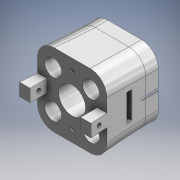
# Autodesk Inventor part: AA008d
Saved by Autodesk Inventor 2017 SP1 (Build 210196100, 196)
## iProperties
Created: 2017-09-28
Part Number: AA008d
Material: ABS Plastic
Document SubType Name: Modeling
Designer: Zach
Density: 1.06 g/cm^3
Appearance: CR White
Author: Zach
Autodesk Inventor part; units mm, degrees
ref_plane "XZ Plane" through (0, 0, 0) normal (0, 1, 0) x (-1, 0, 0)
ref_plane "XY Plane" through (0, 0, 0) normal (0, 0, 1) x (1, 0, 0)
sketch "Sketch1" plane through (0, 0, 0) normal (0, 0, 1) x (1, 0, 0)
  line L0 (0, 0) -> (80, 0)
  line L1 (80, 0) -> (80, 82.6)
  line L2 (80, 82.6) -> (0, 82.6)
  line L3 (0, 82.6) -> (0, 0)
  dimension "d0" = 80
  dimension "d1" = 82.6
  constraints: 8 end point, 2 parallel, 1 horizontal, 1 perpendicular
  measures "d0" distance of L2.end L1.end
  measures "d1" distance of L1.end L0.end
extrude "Extrusion1" add sketch "Sketch1" along normal blind 162.5
sketch "Sketch2" plane through (0, 82.6, 0) normal (0, 1, 0) x (1, 0, 0)
  line L0 (0, -162.5) -> (80, -162.5) projected
  line L1 (-12.5, -162.5) -> (0, -162.5)
  line L2 (80, -162.5) -> (92.5, -162.5)
  line L3 (0, 0) -> (80, 0) projected
  line L4 (0, 0) -> (0, -162.5) projected
  line L5 (80, 0) -> (80, -162.5) projected
  arc A0 (-12.5, -162.5) -> (0, 0) centre (-1199.9534, 10.5733) ccw
  arc A1 (80, 0) -> (92.5, -162.5) centre (1279.9534, 10.5733) ccw
  dimension "d4" = 12.5
  dimension "d5" = 12.5
  dimension "d19" = 1200
  dimension "d20" = 1200
  constraints: 4 end point, 4 point on circle, 2 centre point, 1 collinear, 1 parallel
  measures "d4" distance of L1.start L0.start
  measures "d5" distance of L0.end L2.end
  measures "d19" radius of A0
  measures "d20" radius of A1
extrude "Extrusion2" add sketch "Sketch2" against normal blind 82.6 contours L1 A0 L4 | L5 A1 L2
sketch "Sketch5" plane through (0, 0, 0) normal (0, 0, -1) x (-1, 0, 0)
  line L0 (12.5, 0) -> (-92.5, 0)
  line L1 (-92.5, 0) -> (-92.5, 41.3)
  line L2 (-92.5, 41.3) -> (12.5, 41.3)
  line L3 (12.5, 41.3) -> (12.5, 0)
  point P0 (0, 0)
  point P1 (12.5, 20)
  point P2 (-92.5, 20)
  dimension "d22" = 41.3
  constraints: 8 end point, 2 parallel, 2 point on line, 1 horizontal, 1 horizontal alignment, 1 perpendicular
  measures "d22" distance of L0.end L1.end
extrude "Extrusion4" cut sketch "Sketch5" against normal through all
sketch "Sketch8" plane through (0, 0, 0) normal (1, 0, 0) x (0, 1, 0)
  line L0 (82.6, 162.5) -> (93.8, 162.5)
  line L1 (41.3, 162.5) -> (41.3, 0) projected
  line L2 (82.6, 0) -> (41.3, 0) projected
  arc A0 (93.8, 162.5) -> (82.6, 0) centre (2580.9593, -90.5586) ccw
  line L3 (82.6, 162.5) -> (41.3, 162.5) projected
  line L4 (82.6, 162.5) -> (82.6, 0)
  point P0 (0, 0)
  dimension "d32" = 2500
  dimension "d38" = 11.2
  constraints: 4 end point, 2 point on circle, 1 centre point, 1 horizontal, 1 perpendicular
  measures "d32" radius of A0
  measures "d38" distance of L0.start L0.end
extrude "Extrusion6" add sketch "Sketch8" along normal blind 93 and the other way blind 13 contours L0 A0 L4
sketch "Sketch13" plane through (-13, 82.6, 0) normal (0, -1, 0) x (1, 0, 0)
  arc A0 (13, 0) -> (0.5, 162.5) centre (-1186.9534, -10.5733) ccw projected
  line L0 (0, 162.5) -> (0.5, 162.5) projected
  line L1 (0, 0) -> (0, 162.5) projected
  line L2 (13, 0) -> (0, 0) projected
  arc A1 (105.5, 162.5) -> (93, 0) centre (1292.9534, -10.5733) ccw projected
  line L3 (106, 0) -> (93, 0) projected
  line L4 (106, 162.5) -> (106, 0) projected
  line L5 (105.5, 162.5) -> (106, 162.5) projected
  point P0 (13, 0)
extrude "Extrusion9" cut sketch "Sketch13" against normal through all
fillet "Fillet4" radius 20 2 edges at (-3.5176, 86.9111, 81.8462) (83.5176, 86.9111, 81.8462)
sketch "Sketch38" plane through (0, 0, 162.5) normal (0, 0, 1) x (1, 0, 0)
  line L0 (75, 41.3) -> (5, 41.3)
  circle A0 centre (40, 41.3) radius 4.5
  point P0 (0, 0)
  dimension "d117" = 9
  constraints: 2 end point, 1 centre point, 1 midpoint
  measures "d117" diameter of A0
extrude "Extrusion27" cut sketch "Sketch38" against normal through all
ref_plane "Work Plane14" through (0, 0, 152.5) normal (0, 0, 1) x (1, 0, 0)
sketch "Sketch40" plane through (0, 0, 152.5) normal (0, 0, 1) x (1, 0, 0)
  arc A0 (44.5, 41.3) -> (35.5, 41.3) centre (40, 41.3) ccw projected
  circle A1 centre (40, 41.3) radius 11.5
  point P0 (0, 0)
  dimension "d121" = 23
  constraints: 1 centre point, 1 coincident
  measures "d121" diameter of A1
extrude "Extrusion28" cut sketch "Sketch40" against normal blind 9
ref_plane "Work Plane15" through (0, 0, 61.5) normal (0, 0, 1) x (1, 0, 0)
sketch "Sketch41" plane through (0, 0, 61.5) normal (0, 0, 1) x (1, 0, 0)
  arc A0 (44.5, 41.3) -> (35.5, 41.3) centre (40, 41.3) ccw
  circle A1 centre (40, 41.3) radius 11.5
  point P0 (0, 0)
  dimension "d125" = 23
  constraints: 2 centre point, 2 point on circle, 1 coincident
  measures "d125" diameter of A1
extrude "Extrusion29" cut sketch "Sketch41" against normal blind 9
ref_plane "Work Plane16" through (0, 0, 47.5) normal (0, 0, 1) x (1, 0, 0)
sketch "Sketch43" plane through (0, 0, 47.5) normal (0, 0, 1) x (1, 0, 0)
  arc A0 (44.5, 41.3) -> (35.5, 41.3) centre (40, 41.3) ccw
  line L0 (35.5, 41.3) -> (0, 41.3) construction
  line L1 (0, 62.5933) -> (0, 41.3) construction
  spline S0 degree 3 poles (19.9943, 82.6) (17.3915, 82.6) (14.8137, 82.0916) (9.998, 80.1152) (7.8062, 78.6662) (4.1001, 75.0086) (2.6216, 72.8347) (1.0742, 69.2017) (0.6732, 67.9146) (0.1355, 65.2795) (0, 63.9381) (0, 62.5933) knots 0 0 0 0 0.78083 0.78083 1.561665 1.561665 2.342928 2.342928 2.746314 2.746314 3.149743 3.149743 3.149743 3.149743 construction
  line L2 (60.0057, 82.6) -> (19.9943, 82.6) construction
  spline S1 degree 3 poles (80, 62.5933) (80, 65.2007) (79.4908, 67.7832) (77.5113, 72.6059) (76.0606, 74.8001) (72.4005, 78.5072) (70.2269, 79.985) (66.5969, 81.5295) (65.3131, 81.9291) (62.6848, 82.465) (61.3469, 82.6) (60.0057, 82.6) knots 0 0 0 0 0.782215 0.782215 1.563936 1.563936 2.345071 2.345071 2.747441 2.747441 3.149817 3.149817 3.149817 3.149817 construction
  line L3 (80, 41.3) -> (80, 62.5933) construction
  line L4 (80, 41.3) -> (44.5, 41.3) construction
  line L5 (60.0057, 80.6) -> (19.9943, 80.6)
  line L6 (2, 62.5933) -> (2, 43.3)
  line L7 (2, 43.3) -> (33.8153, 43.3) construction
  arc A1 (46.1847, 43.3) -> (33.8153, 43.3) centre (40, 41.3) ccw construction
  line L8 (46.1847, 43.3) -> (78, 43.3) construction
  line L9 (78, 43.3) -> (78, 62.5933)
  line L10 (2, 43.3) -> (2, 41.3)
  line L11 (78, 43.3) -> (78, 41.3)
  line L12 (44.5, 41.3) -> (78, 41.3)
  line L13 (35.5, 41.3) -> (2, 41.3)
  line L14 (5, 41.3) -> (35.5, 41.3)
  arc A2 (44.5, 41.3) -> (35.5, 41.3) centre (40, 41.3) ccw projected
  spline S2 degree 5 poles (78, 62.5933) (77.9999, 65.4195) (77.4463, 68.2457) (76.3377, 70.927) (73.1281, 75.7135) (68.3466, 78.931) (65.6637, 80.0441) (62.8346, 80.5999) (60.0057, 80.6) knots 0 0 0 0 0 0 0.499755 0.499755 0.499755 1 1 1 1 1 1
  spline S3 degree 5 poles (19.9943, 80.6) (17.1686, 80.5999) (14.3427, 80.0454) (11.6625, 78.9348) (6.8791, 75.7206) (3.666, 70.9361) (2.5549, 68.2521) (2.0001, 65.4227) (2, 62.5933) knots 0 0 0 0 0 0 0.499678 0.499678 0.499678 1 1 1 1 1 1
  dimension "d129" = 2
  constraints: 30 end point, 4 point on circle, 3 centre point, 3 parallel, 2 perpendicular, 2 point on line, 1 collinear, 1 horizontal, 1 horizontal alignment, 18 other
  measures "d129" distance between parallel lines of L3 L9
extrude "Extrusion30" cut sketch "Sketch43" against normal blind 35
sketch "Sketch53" plane through (0, 0, 12.5) normal (0, 0, 1) x (1, 0, 0)
  arc A0 (44.5, 41.3) -> (35.5, 41.3) centre (40, 41.3) ccw projected
  circle A1 centre (40, 41.3) radius 2.5 construction
  line L0 (44.5, 41.3) -> (42.5, 41.3)
  line L1 (35.5, 41.3) -> (37.5, 41.3)
  arc A2 (42.5, 41.3) -> (37.5, 41.3) centre (40, 41.3) ccw
  point P0 (0, 0)
  dimension "d163" = 5
  constraints: 4 end point, 4 point on circle, 2 centre point, 1 coincident, 1 concentric, 1 horizontal, 1 point on line
  measures "d163" diameter of A1
extrude "Extrusion39" add sketch "Sketch53" against normal blind 2
sketch "Sketch54" plane through (0, 0, 0) normal (0, 0, -1) x (-1, 0, 0)
  arc A0 (-35.5, 41.3) -> (-44.5, 41.3) centre (-40, 41.3) ccw projected
  circle A1 centre (-40, 41.3) radius 16.5
  point P0 (0, 0)
  dimension "d166" = 33
  constraints: 1 centre point, 1 coincident
  measures "d166" diameter of A1
extrude "Extrusion40" cut sketch "Sketch54" against normal blind 7.5
sketch "Sketch55" plane through (0, 0, 12.5) normal (0, 0, 1) x (1, 0, 0)
  arc A0 (42.5, 41.3) -> (37.5, 41.3) centre (40, 41.3) ccw projected
  circle A1 centre (40, 49.8) radius 2
  point P0 (0, 0)
  dimension "d169" = 4
  dimension "d170" = 8.5
  constraints: 1 centre point, 1 vertical alignment
  measures "d169" diameter of A1
  measures "d170" distance of A0.centre A1.centre
extrude "Extrusion41" cut sketch "Sketch55" against normal through all
sketch "Sketch56" plane through (0, 0, 12.5) normal (0, 0, 1) x (1, 0, 0)
  circle A0 centre (40, 49.8) radius 2 projected
  circle A1 centre (40, 49.8) radius 3.5
  point P0 (0, 0)
  dimension "d173" = 7
  constraints: 1 centre point, 1 coincident
  measures "d173" diameter of A1
extrude "Extrusion42" cut sketch "Sketch56" against normal blind 3
sketch "Sketch63" plane through (0, 0, 47.5) normal (0, 0, -1) x (-1, 0, 0)
  circle A0 centre (-40, 41.3) radius 16 construction
  arc A1 (-24, 41.3) -> (-56, 41.3) centre (-40, 41.3) ccw
  arc A2 (-35.5, 41.3) -> (-44.5, 41.3) centre (-40, 41.3) ccw construction
  line L0 (-2, 41.3) -> (-35.5, 41.3) construction
  line L1 (-2, 41.3) -> (-2, 62.5933) projected
  spline S0 degree 5 poles (-2, 62.5933) (-2.0001, 65.4227) (-2.5549, 68.2521) (-3.666, 70.9361) (-6.8791, 75.7206) (-11.6625, 78.9348) (-14.3427, 80.0454) (-17.1686, 80.5999) (-19.9943, 80.6) knots 0 0 0 0 0 0 0.500322 0.500322 0.500322 1 1 1 1 1 1 projected
  line L2 (-19.9943, 80.6) -> (-60.0057, 80.6) projected
  spline S1 degree 5 poles (-60.0057, 80.6) (-62.8346, 80.5999) (-65.6637, 80.0441) (-68.3466, 78.931) (-73.1281, 75.7135) (-76.3377, 70.927) (-77.4463, 68.2457) (-77.9999, 65.4195) (-78, 62.5933) knots 0 0 0 0 0 0 0.500245 0.500245 0.500245 1 1 1 1 1 1 projected
  line L3 (-78, 62.5933) -> (-78, 41.3) projected
  line L4 (-44.5, 41.3) -> (-78, 41.3) construction
  line L5 (-78, 41.3) -> (-56, 41.3)
  line L6 (-24, 41.3) -> (-2, 41.3)
  point P0 (0, 0)
  dimension "d207" = 32
  constraints: 4 end point, 4 point on circle, 2 centre point, 2 collinear, 1 coincident, 1 concentric, 1 horizontal alignment, 2 other
  measures "d207" diameter of A0
extrude "Extrusion49" add sketch "Sketch63" along normal blind 35
sketch "Sketch65" plane through (0, 0, 0) normal (0, 0, -1) x (-1, 0, 0)
  circle A0 centre (-40, 71.3) radius 2.5
  arc A1 (-35.5, 41.3) -> (-44.5, 41.3) centre (-40, 41.3) ccw projected
  point P0 (0, 0)
  dimension "d214" = 5
  dimension "d215" = 30
  constraints: 1 centre point, 1 vertical alignment
  measures "d214" diameter of A0
  measures "d215" distance of A1.centre A0.centre
extrude "Extrusion51" cut sketch "Sketch65" against normal blind 75
sketch "Sketch66" plane through (0, 0, 0) normal (0, 0, -1) x (-1, 0, 0)
  circle A0 centre (-40, 71.3) radius 6.5
  circle A1 centre (-40, 71.3) radius 2.5 projected
  point P0 (0, 0)
  dimension "d218" = 13
  constraints: 1 centre point, 1 coincident
  measures "d218" diameter of A0
extrude "Extrusion52" cut sketch "Sketch66" against normal blind 35 contours A0 | A1
mirror "Mirror1" about plane through (92.5, 41.3, 0) normal (0, -1, 0)
sketch "Sketch69" plane through (0, 0, 0) normal (0, 1, 0) x (-1, 0, 0)
  line L0 (-35.5, 143.5) -> (-44.5, 143.5) projected
  line L1 (-51.5, 143.5) -> (-28.5, 143.5) projected
  line L2 (-44.5, 152.5) -> (-35.5, 152.5) projected
  line L3 (-28.5, 61.5) -> (-51.5, 61.5) projected
  line L4 (-44.5, 61.5) -> (-35.5, 61.5) projected
  line L5 (-35.5, 52.5) -> (-44.5, 52.5) projected
  line L6 (-51.5, 61.5) -> (-28.5, 61.5)
  line L7 (-28.5, 61.5) -> (-28.5, 52.5)
  line L8 (-28.5, 52.5) -> (-51.5, 52.5)
  line L9 (-51.5, 52.5) -> (-51.5, 61.5)
  line L10 (-51.5, 143.5) -> (-28.5, 143.5)
  line L11 (-28.5, 143.5) -> (-28.5, 152.5)
  line L12 (-28.5, 152.5) -> (-51.5, 152.5)
  line L13 (-51.5, 152.5) -> (-51.5, 143.5)
  point P0 (0, 0)
  point P1 (-40, 52.5)
  point P2 (-40, 152.5)
  constraints: 16 end point, 4 midpoint, 4 parallel, 2 horizontal, 2 perpendicular, 1 point on line
extrude "Extrusion54" cut sketch "Sketch69" along normal blind 41.5 and the other way blind 15
sketch "Sketch71" plane through (0, 0, 0) normal (0, 0, -1) x (-1, 0, 0)
  line L0 (-17.5, 18.8) -> (-62.5, 18.8) construction
  line L1 (-62.5, 18.8) -> (-62.5, 63.8) construction
  line L2 (-62.5, 63.8) -> (-17.5, 63.8) construction
  line L3 (-17.5, 63.8) -> (-17.5, 18.8) construction
  circle A0 centre (-40, 41.3) radius 4.5 construction
  circle A1 centre (-17.5, 18.8) radius 2.5
  circle A2 centre (-62.5, 18.8) radius 2.5
  circle A3 centre (-62.5, 63.8) radius 2.5
  circle A4 centre (-17.5, 63.8) radius 2.5
  point P0 (0, 0)
  point P1 (-17.5, 41.3)
  point P2 (-40, 18.8)
  dimension "d229" = 45
  dimension "d230" = 45
  dimension "d231" = 5
  dimension "d232" = 5
  dimension "d233" = 5
  dimension "d234" = 5
  constraints: 8 end point, 4 centre point, 4 coincident, 2 midpoint, 2 parallel, 1 horizontal, 1 horizontal alignment, 1 perpendicular, 1 vertical alignment
  measures "d229" distance of L1.end L2.end
  measures "d230" distance of L0.end L1.end
  measures "d231" diameter of A1
  measures "d232" diameter of A2
  measures "d233" diameter of A3
  measures "d234" diameter of A4
extrude "Extrusion56" cut sketch "Sketch71" against normal through all
sketch "Sketch72" plane through (0, 0, 162.5) normal (0, 0, 1) x (1, 0, 0)
  circle A0 centre (40, 41.3) radius 4.5 construction
  line L0 (-12.5, 8.6096) -> (-12.5, 73.9904) construction
  spline S0 degree 3 poles (-12.5, 8.6096) (-12.5, 6.0114) (-11.9936, 3.4396) (-10.0229, -1.3365) (-8.5896, -3.495) (-4.9699, -7.1453) (-2.8204, -8.5984) (0.7865, -10.1299) (2.0756, -10.5292) (4.7184, -11.0654) (6.0655, -11.2) (7.4159, -11.2) knots 0 0 0 0 0.779465 0.779465 1.550261 1.550261 2.321978 2.321978 2.725865 2.725865 3.130971 3.130971 3.130971 3.130971 construction
  line L1 (7.4159, -11.2) -> (72.5841, -11.2) construction
  spline S1 degree 3 poles (72.5841, -11.2) (75.222, -11.2) (77.8346, -10.6862) (82.6695, -8.6891) (84.8494, -7.2416) (88.5077, -3.6012) (89.955, -1.4536) (91.9757, 3.3497) (92.5, 5.9658) (92.5, 8.6096) knots 0 0 0 0 0.791372 0.791372 1.569712 1.569712 2.340306 2.340306 3.13363 3.13363 3.13363 3.13363 construction
  line L2 (92.5, 73.9904) -> (92.5, 8.6096) construction
  spline S2 degree 3 poles (72.5841, 93.8) (75.222, 93.8) (77.8346, 93.2862) (82.6695, 91.2891) (84.8494, 89.8416) (88.5077, 86.2012) (89.955, 84.0536) (91.9757, 79.2503) (92.5, 76.6342) (92.5, 73.9904) knots 0 0 0 0 0.791372 0.791372 1.569712 1.569712 2.340306 2.340306 3.13363 3.13363 3.13363 3.13363 construction
  line L3 (7.4159, 93.8) -> (72.5841, 93.8) construction
  spline S3 degree 3 poles (-12.5, 73.9904) (-12.5, 76.5886) (-11.9936, 79.1604) (-10.0229, 83.9365) (-8.5896, 86.095) (-4.9699, 89.7453) (-2.8204, 91.1984) (0.7865, 92.7299) (2.0756, 93.1292) (4.7184, 93.6654) (6.0655, 93.8) (7.4159, 93.8) knots 0 0 0 0 0.779465 0.779465 1.550261 1.550261 2.321978 2.321978 2.725865 2.725865 3.130971 3.130971 3.130971 3.130971 construction
  circle A1 centre (17.5, 63.8) radius 10
  circle A2 centre (62.5, 63.8) radius 10
  circle A3 centre (62.5, 18.8) radius 10
  circle A4 centre (17.5, 18.8) radius 10
  circle A5 centre (62.5, 18.8) radius 2.5 projected
  circle A6 centre (62.5, 63.8) radius 2.5 projected
  circle A7 centre (17.5, 63.8) radius 2.5 projected
  circle A8 centre (17.5, 18.8) radius 2.5 projected
  point P0 (0, 0)
  dimension "d237" = 20
  dimension "d238" = 20
  dimension "d239" = 20
  dimension "d240" = 20
  constraints: 8 end point, 5 centre point, 4 coincident, 8 other
  measures "d237" diameter of A1
  measures "d238" diameter of A2
  measures "d239" diameter of A3
  measures "d240" diameter of A4
extrude "Extrusion57" cut sketch "Sketch72" against normal blind 157.5 contours A1 | A2 | A3 | A4 | A5 | A6 | A7 | A8
sketch "Sketch77" plane through (40, 41.3, 12.5) normal (0, 0, 1) x (1, 0, 0)
  circle A0 centre (0, 0) radius 16 projected
  line L0 (0, -16) -> (-50, -16)
  line L1 (-50, -16) -> (-50, 16)
  line L2 (-50, 16) -> (0, 16)
  line L3 (0, 16) -> (0, -16)
  point P0 (-40, -41.3)
  dimension "d253" = 50
  constraints: 8 end point, 2 coincident, 2 parallel, 2 point on circle, 2 vertical alignment, 1 centre point, 1 horizontal, 1 midpoint, 1 perpendicular
  measures "d253" distance of L1.end L2.end
extrude "Extrusion61" cut sketch "Sketch77" along normal blind 6 contours L3 A0 | A0 L0 L1 L2 picked at (-2.4785, 4.7224)
sketch "Sketch76" plane through (40, 41.3, 47.5) normal (0, 0, -1) x (-1, 0, 0)
  circle A0 centre (-22.5, -22.5) radius 10 projected
  circle A1 centre (22.5, 22.5) radius 10 projected
  circle A2 centre (-22.5, 22.5) radius 10 projected
  circle A3 centre (22.5, -22.5) radius 10 projected
  line L0 (-52.5, 32.6904) -> (-52.5, -32.6904) projected
  spline S0 degree 7 poles (-32.5841, 52.5) (-33.3627, 52.5) (-34.1548, 52.4652) (-34.9579, 52.3933) (-35.7692, 52.2823) (-36.5854, 52.1305) (-37.403, 51.9365) (-38.4905, 51.6204) (-38.7626, 51.5364) (-39.0343, 51.4477) (-39.3054, 51.354) (-39.5759, 51.2555) (-39.8454, 51.1522) (-41.1893, 50.6105) (-42.2483, 50.0989) (-43.281, 49.5093) (-44.2775, 48.8434) (-45.2278, 48.1054) (-46.1232, 47.3015) (-47.7481, 45.6204) (-48.4837, 44.7489) (-49.1573, 43.8314) (-49.7641, 42.8755) (-50.301, 41.8899) (-50.7669, 40.883) (-51.559, 38.8386) (-51.8845, 37.8008) (-52.1388, 36.7585) (-52.3238, 35.7196) (-52.4429, 34.6914) (-52.5, 33.68) (-52.5, 32.6904) knots 0 0 0 0 0 0 0 0 0.191534 0.191534 0.191534 0.191534 0.191534 0.191534 0.255547 0.255547 0.255547 0.255547 0.255547 0.255547 0.5119 0.5119 0.5119 0.5119 0.5119 0.5119 0.755356 0.755356 0.755356 0.755356 0.755356 0.755356 1 1 1 1 1 1 1 1 projected
  line L1 (32.5841, 52.5) -> (-32.5841, 52.5) projected
  spline S1 degree 7 poles (52.5, 32.6904) (52.5, 33.68) (52.4429, 34.6914) (52.3238, 35.7196) (52.1388, 36.7585) (51.8845, 37.8008) (51.559, 38.8386) (50.7669, 40.8829) (50.3011, 41.8897) (49.7642, 42.8753) (49.1575, 43.8311) (48.484, 44.7486) (47.7485, 45.62) (46.1237, 47.3011) (45.2283, 48.105) (44.278, 48.843) (43.2815, 49.5089) (42.2488, 50.0986) (41.1898, 50.6102) (39.8459, 51.152) (39.5764, 51.2553) (39.306, 51.3538) (39.0348, 51.4475) (38.7631, 51.5363) (38.491, 51.6203) (37.4035, 51.9364) (36.5858, 52.1304) (35.7695, 52.2823) (34.9581, 52.3933) (34.1549, 52.4652) (33.3628, 52.5) (32.5841, 52.5) knots 0 0 0 0 0 0 0 0 0.244644 0.244644 0.244644 0.244644 0.244644 0.244644 0.488082 0.488082 0.488082 0.488082 0.488082 0.488082 0.744435 0.744435 0.744435 0.744435 0.744435 0.744435 0.808449 0.808449 0.808449 0.808449 0.808449 0.808449 1 1 1 1 1 1 1 1 projected
  line L2 (52.5, -32.6904) -> (52.5, 32.6904) projected
  spline S2 degree 7 poles (52.5, -32.6904) (52.5, -33.68) (52.4429, -34.6914) (52.3238, -35.7196) (52.1388, -36.7585) (51.8845, -37.8008) (51.559, -38.8386) (50.7669, -40.8829) (50.3011, -41.8897) (49.7642, -42.8753) (49.1575, -43.8311) (48.484, -44.7486) (47.7485, -45.62) (46.1237, -47.3011) (45.2283, -48.105) (44.278, -48.843) (43.2815, -49.5089) (42.2488, -50.0986) (41.1898, -50.6102) (39.8459, -51.152) (39.5764, -51.2553) (39.306, -51.3538) (39.0348, -51.4475) (38.7631, -51.5363) (38.491, -51.6203) (37.4035, -51.9364) (36.5858, -52.1304) (35.7695, -52.2823) (34.9581, -52.3933) (34.1549, -52.4652) (33.3628, -52.5) (32.5841, -52.5) knots 0 0 0 0 0 0 0 0 0.244644 0.244644 0.244644 0.244644 0.244644 0.244644 0.488082 0.488082 0.488082 0.488082 0.488082 0.488082 0.744435 0.744435 0.744435 0.744435 0.744435 0.744435 0.808449 0.808449 0.808449 0.808449 0.808449 0.808449 1 1 1 1 1 1 1 1 projected
  line L3 (32.5841, -52.5) -> (-32.5841, -52.5) projected
  spline S3 degree 7 poles (-32.5841, -52.5) (-33.3627, -52.5) (-34.1548, -52.4652) (-34.9579, -52.3933) (-35.7692, -52.2823) (-36.5854, -52.1305) (-37.403, -51.9365) (-38.4905, -51.6204) (-38.7626, -51.5364) (-39.0343, -51.4477) (-39.3054, -51.354) (-39.5759, -51.2555) (-39.8454, -51.1522) (-41.1893, -50.6105) (-42.2483, -50.0989) (-43.281, -49.5093) (-44.2775, -48.8434) (-45.2278, -48.1054) (-46.1232, -47.3015) (-47.7481, -45.6204) (-48.4837, -44.7489) (-49.1573, -43.8314) (-49.7641, -42.8755) (-50.301, -41.8899) (-50.7669, -40.883) (-51.559, -38.8386) (-51.8845, -37.8008) (-52.1388, -36.7585) (-52.3238, -35.7196) (-52.4429, -34.6914) (-52.5, -33.68) (-52.5, -32.6904) knots 0 0 0 0 0 0 0 0 0.191534 0.191534 0.191534 0.191534 0.191534 0.191534 0.255547 0.255547 0.255547 0.255547 0.255547 0.255547 0.5119 0.5119 0.5119 0.5119 0.5119 0.5119 0.755356 0.755356 0.755356 0.755356 0.755356 0.755356 1 1 1 1 1 1 1 1 projected
  circle A4 centre (0, 0) radius 4.5 projected
  line L4 (-52.5, 32.6904) -> (-52.5, -32.6904) projected
  line L5 (-52.5, -7.5) -> (-30, -7.5)
  line L6 (-30, -7.5) -> (-30, 7.5)
  line L7 (-30, 7.5) -> (-52.5, 7.5)
  line L8 (-52.5, 7.5) -> (-52.5, -7.5)
  line L9 (30, 7.5) -> (52.5, 7.5)
  line L10 (52.5, 7.5) -> (52.5, -7.5)
  line L11 (52.5, -7.5) -> (30, -7.5)
  line L12 (30, -7.5) -> (30, 7.5)
  point P0 (40, -41.3)
  point P1 (-30, 0)
  dimension "d256" = 15
  dimension "d257" = 30
  dimension "d300" = 30
  constraints: 16 end point, 4 parallel, 3 horizontal alignment, 2 horizontal, 2 perpendicular, 2 point on line, 1 midpoint, 4 other
  measures "d256" distance of L6.end L5.end
  measures "d257" distance from line of A4.centre L6
  measures "d300" distance from line of L12 A4.centre
extrude "Extrusion62" cut sketch "Sketch76" against normal through all contours S0 L1 S1 L2 L9 L12 L11 S2 L3 S3 L0 L5 L6 L7
ref_plane "Work Plane20" through (40, 41.3, 67.5) normal (0, 0, 1) x (1, 0, 0)
sketch "Sketch78" plane through (40, 41.3, 67.5) normal (0, 0, 1) x (1, 0, 0)
  line L0 (30, -7.5) -> (52.5, -7.5) projected
  line L1 (52.5, 7.5) -> (52.5, -7.5) projected
  line L2 (52.5, 7.5) -> (30, 7.5) projected
  line L3 (30, 7.5) -> (30, -7.5) projected
  line L4 (-30, 7.5) -> (-52.5, 7.5) projected
  line L5 (-52.5, -7.5) -> (-52.5, 7.5) projected
  line L6 (-52.5, -7.5) -> (-30, -7.5) projected
  line L7 (-30, -7.5) -> (-30, 7.5) projected
  point P0 (-40, -41.3)
extrude "Extrusion63" cut sketch "Sketch78" along normal through all
sketch "Sketch79" plane through (70, 33.8, 47.5) normal (-1, 0, 0) x (0, 0, 1)
  circle A0 centre (10, 7.5) radius 2.5
  line L0 (20, 0) -> (20, 15) projected
  line L1 (0, -15.9972) -> (0, 30.9972) projected
  point P0 (-47.5, -33.8)
  point P1 (20, 7.5)
  dimension "d263" = 5
  dimension "d264" = 10
  constraints: 1 centre point, 1 horizontal alignment, 1 midpoint
  measures "d263" diameter of A0
  measures "d264" distance from line of A0.centre L1
extrude "Extrusion64" cut sketch "Sketch79" along normal through all both and the other way through all
ref_plane "Work Plane21" through (0, 0, 17) normal (0, 0, -1) x (-1, 0, 0)
sketch "Sketch81" plane through (0, 0, 17) normal (0, 0, -1) x (-1, 0, 0)
  circle A0 centre (-40, 41.3) radius 2.5 projected
  line L0 (-40, 57.3) -> (-82.4959, 57.3)
  line L1 (-40, 25.3) -> (-82.4959, 25.3)
  line L2 (-82.4959, 57.3) -> (-82.4959, 25.3)
  line L3 (-82.4959, 48.8) -> (-82.4959, 33.8) projected
  line L4 (-40, 57.3) -> (-40, 25.3)
  point P0 (0, 0)
  point P1 (-82.4959, 41.3)
  constraints: 8 end point, 2 horizontal, 2 midpoint, 2 vertical
extrude "Extrusion65" cut sketch "Sketch81" against normal blind 6 contours L4 A0 | A0 L4 L1 L2 L0 picked at (-41.4604, 40.8266)
sketch "Sketch82" plane through (0, 0, 0) normal (0, 0, -1) x (-1, 0, 0)
  circle A0 centre (-40, 41.3) radius 2.5 projected
  line L0 (-79, 29.8) -> (-55, 29.8)
  line L1 (-55, 29.8) -> (-55, 52.8)
  line L2 (-55, 52.8) -> (-79, 52.8)
  line L3 (-79, 52.8) -> (-79, 29.8)
  line L4 (-67, 29.8) -> (-67, 52.8)
  point P0 (0, 0)
  point P1 (-67, 41.3)
  dimension "d272" = 27
  dimension "d273" = 23
  dimension "d274" = 24
  constraints: 10 end point, 3 midpoint, 2 parallel, 1 horizontal, 1 horizontal alignment, 1 perpendicular
  measures "d272" distance from line of A0.centre L4
  measures "d273" distance of L2.end L0.start
  measures "d274" distance of L0.start L0.end
extrude "Extrusion66" cut sketch "Sketch82" against normal blind 5 contours L3 L2 L4 L0 | L4 L2 L1 L0
sketch "Sketch83" plane through (0, 0, 5) normal (0, 0, -1) x (-1, 0, 0)
  circle A0 centre (-67, 41.3) radius 6.5
  circle A1 centre (-40, 41.3) radius 2.5 projected
  point P0 (0, 0)
  dimension "d277" = 13
  dimension "d278" = 27
  constraints: 1 centre point, 1 horizontal alignment
  measures "d277" diameter of A0
  measures "d278" distance of A1.centre A0.centre
extrude "Extrusion67" cut sketch "Sketch83" against normal blind 24 contours A0
ref_plane "Work Plane22" through (67, 0, 0) normal (1, 0, 0) x (0, 1, 0)
sketch "Sketch86" plane through (0, 0, 5) normal (0, 0, -1) x (-1, 0, 0)
  line L0 (-53.5, 42.8) -> (-80.5, 42.8)
  line L1 (-80.5, 42.8) -> (-80.5, 39.8)
  line L2 (-80.5, 39.8) -> (-53.5, 39.8)
  line L3 (-53.5, 39.8) -> (-53.5, 42.8)
  circle A0 centre (-67, 41.3) radius 6.5 projected
  point P0 (0, 0)
  point P1 (-53.5, 41.3)
  point P2 (-67, 39.8)
  dimension "d284" = 27
  dimension "d285" = 3
  constraints: 8 end point, 2 midpoint, 2 parallel, 1 horizontal, 1 horizontal alignment, 1 perpendicular, 1 vertical alignment
  measures "d284" distance of L2.end L1.end
  measures "d285" distance of L1.end L0.end
extrude "Extrusion69" cut sketch "Sketch86" along normal through all contours L3 L2 A0 L0 | A0 L2 L0 | A0 L2 L1 L0
sketch "Sketch87" plane through (0, 0, 5) normal (0, 0, -1) x (-1, 0, 0)
  line L0 (-75.5, 43.3) -> (-78.5, 43.3)
  line L1 (-78.5, 43.3) -> (-78.5, 39.3)
  line L2 (-78.5, 39.3) -> (-75.5, 39.3)
  line L3 (-75.5, 39.3) -> (-75.5, 43.3)
  circle A0 centre (-67, 41.3) radius 6.5 projected
  point P0 (0, 0)
  point P1 (-75.5, 41.3)
  dimension "d288" = 3
  dimension "d289" = 4
  dimension "d290" = 8.5
  constraints: 8 end point, 2 parallel, 1 horizontal, 1 horizontal alignment, 1 midpoint, 1 perpendicular
  measures "d288" distance of L2.end L1.end
  measures "d289" distance of L1.end L0.end
  measures "d290" distance from line of A0.centre L3
extrude "Extrusion70" cut sketch "Sketch87" against normal blind 2 contours L3 L2 L1 L0
sketch "Sketch88" plane through (40, 41.3, 47.5) normal (0, 0, 1) x (1, 0, 0)
  circle A0 centre (27, 0) radius 6.5 projected
  circle A1 centre (27, 0) radius 3
  point P0 (-40, -41.3)
  dimension "d293" = 6
  constraints: 1 centre point, 1 coincident
  measures "d293" diameter of A1
extrude "Extrusion71" cut sketch "Sketch88" against normal through all contours A1
sketch "Sketch89" plane through (0, 0, 0) normal (0, 0, -1) x (-1, 0, 0)
  line L0 (-79, 39.8) -> (-80, 39.8) projected
  line L1 (-80, 20.0067) -> (-80, 39.8) construction
  spline S0 degree 7 poles (-80, 20.0067) (-80, 18.9899) (-79.9398, 17.9489) (-79.8141, 16.8891) (-79.6185, 15.8172) (-79.3494, 14.741) (-79.0048, 13.6696) (-78.1647, 11.5558) (-77.6693, 10.5135) (-77.0984, 9.4944) (-76.4534, 8.5082) (-75.7381, 7.5642) (-74.9582, 6.6711) (-73.2833, 5.0007) (-72.3883, 4.2234) (-71.4428, 3.511) (-70.4554, 2.8691) (-69.4355, 2.3014) (-68.3928, 1.8094) (-66.2875, 0.9794) (-65.2251, 0.6403) (-64.1584, 0.3755) (-63.096, 0.183) (-62.0456, 0.0593) (-61.0138, 0) (-60.0057, 0) knots 0 0 0 0 0 0 0 0 0.250646 0.250646 0.250646 0.250646 0.250646 0.250646 0.501009 0.501009 0.501009 0.501009 0.501009 0.501009 0.751364 0.751364 0.751364 0.751364 0.751364 0.751364 1 1 1 1 1 1 1 1 projected
  line L2 (-60.0057, 0) -> (-19.9943, 0) projected
  spline S1 degree 7 poles (-19.9943, 0) (-18.9984, 0) (-17.9793, 0.0579) (-16.9421, 0.1785) (-15.8929, 0.3662) (-14.8392, 0.6244) (-13.7894, 0.955) (-11.6907, 1.7709) (-10.6424, 2.2597) (-9.6165, 2.8249) (-8.6229, 3.465) (-7.6711, 4.1764) (-6.7698, 4.9535) (-5.0827, 6.625) (-4.2968, 7.5194) (-3.5759, 8.4653) (-2.9257, 9.4542) (-2.35, 10.4765) (-1.8506, 11.5224) (-1.0035, 13.6439) (-0.656, 14.7195) (-0.3846, 15.8001) (-0.1874, 16.8764) (-0.0607, 17.9406) (0, 18.9859) (0, 20.0067) knots 0 0 0 0 0 0 0 0 0.245635 0.245635 0.245635 0.245635 0.245635 0.245635 0.496987 0.496987 0.496987 0.496987 0.496987 0.496987 0.748353 0.748353 0.748353 0.748353 0.748353 0.748353 1 1 1 1 1 1 1 1 projected
  line L3 (0, 62.5933) -> (0, 20.0067) projected
  spline S2 degree 7 poles (-19.9943, 82.6) (-18.9984, 82.6) (-17.9793, 82.5421) (-16.9421, 82.4215) (-15.8929, 82.2338) (-14.8392, 81.9756) (-13.7894, 81.645) (-11.6907, 80.8291) (-10.6424, 80.3403) (-9.6165, 79.7751) (-8.6229, 79.135) (-7.6711, 78.4236) (-6.7698, 77.6465) (-5.0827, 75.975) (-4.2968, 75.0806) (-3.5759, 74.1347) (-2.9257, 73.1458) (-2.35, 72.1235) (-1.8506, 71.0776) (-1.0035, 68.9561) (-0.656, 67.8805) (-0.3846, 66.7999) (-0.1874, 65.7236) (-0.0607, 64.6594) (0, 63.6141) (0, 62.5933) knots 0 0 0 0 0 0 0 0 0.245635 0.245635 0.245635 0.245635 0.245635 0.245635 0.496987 0.496987 0.496987 0.496987 0.496987 0.496987 0.748353 0.748353 0.748353 0.748353 0.748353 0.748353 1 1 1 1 1 1 1 1 projected
  line L4 (-60.0057, 82.6) -> (-19.9943, 82.6) projected
  spline S3 degree 7 poles (-80, 62.5933) (-80, 63.6101) (-79.9398, 64.6511) (-79.8141, 65.7109) (-79.6185, 66.7828) (-79.3494, 67.859) (-79.0048, 68.9304) (-78.1647, 71.0442) (-77.6693, 72.0865) (-77.0984, 73.1056) (-76.4534, 74.0918) (-75.7381, 75.0358) (-74.9582, 75.9289) (-73.2833, 77.5993) (-72.3883, 78.3766) (-71.4428, 79.089) (-70.4554, 79.7309) (-69.4355, 80.2986) (-68.3928, 80.7906) (-66.2875, 81.6206) (-65.2251, 81.9597) (-64.1584, 82.2245) (-63.096, 82.417) (-62.0456, 82.5407) (-61.0138, 82.6) (-60.0057, 82.6) knots 0 0 0 0 0 0 0 0 0.250646 0.250646 0.250646 0.250646 0.250646 0.250646 0.501009 0.501009 0.501009 0.501009 0.501009 0.501009 0.751364 0.751364 0.751364 0.751364 0.751364 0.751364 1 1 1 1 1 1 1 1 projected
  line L5 (-80, 42.8) -> (-80, 62.5933) construction
  line L6 (-80, 42.8) -> (-79, 42.8) projected
  line L7 (-79, 42.8) -> (-79, 52.8) construction
  line L8 (-79, 52.8) -> (-55, 52.8) construction
  line L9 (-55, 52.8) -> (-55, 48.1739) construction
  arc A0 (-55, 34.4261) -> (-55, 48.1739) centre (-40, 41.3) ccw construction
  line L10 (-55, 34.4261) -> (-55, 29.8) construction
  line L11 (-55, 29.8) -> (-79, 29.8) construction
  line L12 (-79, 29.8) -> (-79, 39.8) construction
  circle A1 centre (-40, 71.3) radius 6.5 projected
  circle A2 centre (-40, 11.3) radius 6.5 projected
  circle A3 centre (-17.5, 63.8) radius 2.5 projected
  circle A4 centre (-62.5, 18.8) radius 2.5 projected
  circle A5 centre (-17.5, 18.8) radius 2.5 projected
  circle A6 centre (-62.5, 63.8) radius 2.5 projected
  line L13 (-80, 42.8) -> (-80, 62.5933) projected
  line L14 (-80, 62.5933) -> (-80, 20.0067)
  arc A7 (-55, 34.4261) -> (-55, 48.1739) centre (-40, 41.3) ccw projected
  line L15 (-40, 57.8) -> (-79, 57.8)
  line L16 (-79, 57.8) -> (-79, 24.8)
  line L17 (-79, 24.8) -> (-40, 24.8)
  arc A8 (-40, 24.8) -> (-40, 57.8) centre (-40, 41.3) ccw
  point P0 (0, 0)
  constraints: 8 end point, 6 point on circle, 3 tangent, 3 vertical alignment, 1 centre point, 1 collinear, 1 horizontal, 1 point on line, 4 other
extrude "Extrusion72" add sketch "Sketch89" along normal blind 15 contours L16 L17 A7 L15 L6 L13 S3 L4 S2 L3 S1 L2 S0 L14 L0 | L0 L14 L6 L16
sketch "Sketch90" plane through (0, 0, 5) normal (0, 0, -1) x (-1, 0, 0)
  line L0 (-80.0545, 39.8) -> (-80.0545, 42.8) projected
  line L1 (-79, 29.8) -> (-79, 39.8) projected
  line L2 (-80.0545, 42.8) -> (-79, 42.8)
  line L3 (-79, 42.8) -> (-79, 39.8)
  line L4 (-79, 39.8) -> (-80.0545, 39.8)
  line L5 (-80.0545, 39.8) -> (-80.0545, 42.8)
  point P0 (0, 0)
  constraints: 8 end point, 2 parallel, 1 horizontal, 1 perpendicular
extrude "Extrusion73" cut sketch "Sketch90" along normal through all
sketch "Sketch91" plane through (0, 0, 23) normal (0, 0, -1) x (-1, 0, 0)
  circle A0 centre (-67, 41.3) radius 3 projected
  circle A1 centre (-67, 41.3) radius 6.5 projected
  arc A2 (-54.9007, 25.3) -> (-70.0993, 25.3) centre (-62.5, 18.8) ccw projected
  line L0 (-40, 25.3) -> (-54.9007, 25.3) projected
  arc A3 (-40, 57.3) -> (-40, 25.3) centre (-40, 41.3) ccw projected
  line L1 (-54.9007, 57.3) -> (-40, 57.3) projected
  arc A4 (-70.0993, 57.3) -> (-54.9007, 57.3) centre (-62.5, 63.8) ccw projected
  line L2 (-80.4232, 57.3) -> (-70.0993, 57.3) projected
  line L3 (-80.4232, 25.3) -> (-80.4232, 57.3) projected
  line L4 (-70.0993, 25.3) -> (-80.4232, 25.3) projected
  circle A5 centre (-67, 41.3) radius 18.5
  point P0 (0, 0)
  dimension "d301" = 37
  constraints: 1 centre point, 1 coincident
  measures "d301" diameter of A5
extrude "Extrusion74" cut sketch "Sketch91" along normal blind 6 contours A5 L4 A2 | A2 L4 A5 L3 L2 A4 A3 | A3 A5 | A5 L3 | A4 L2 A5
equation "\"d5\" = d4"
body "Solid1"
